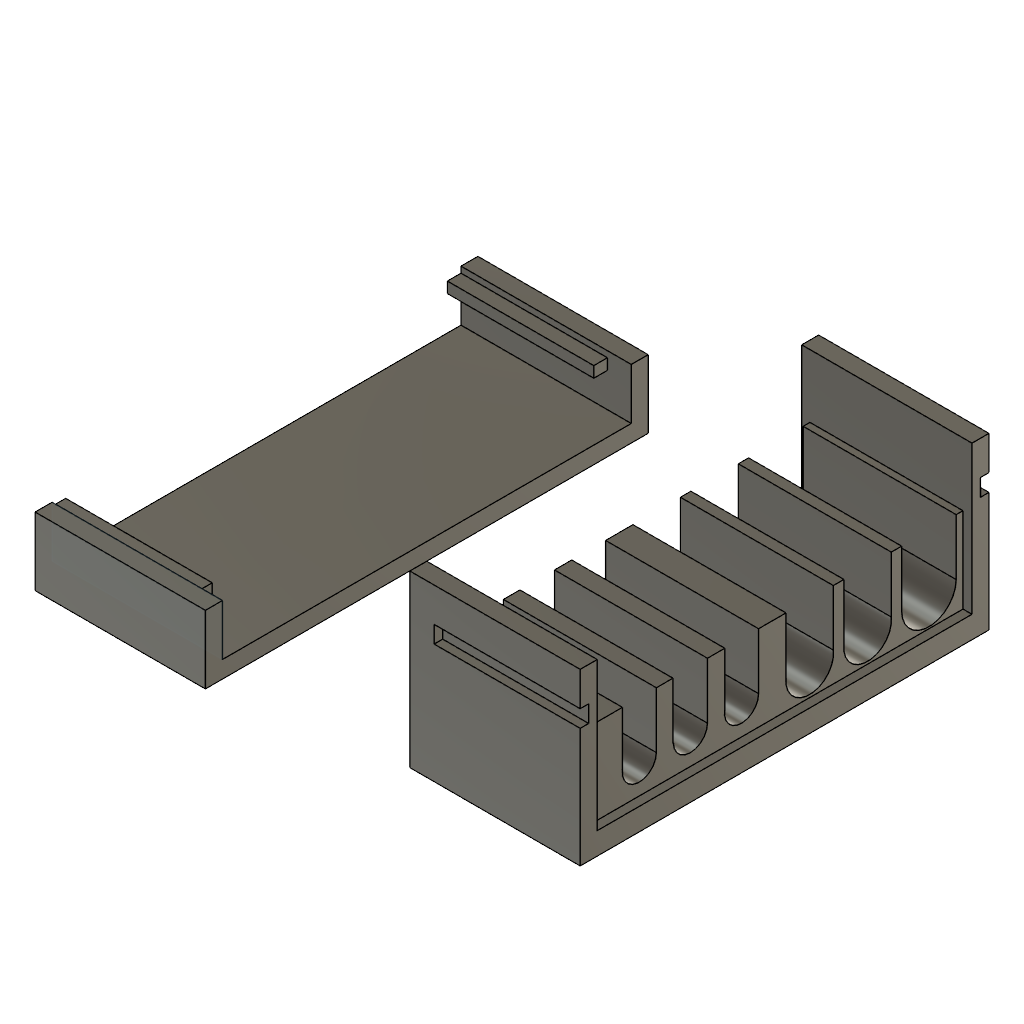
cable management clamp (Autodesk Fusion 360 design; units mm, degrees)
part number: 2026-09-18-19-42-44-531
Autodesk Fusion 360 part; units mm, degrees
note: some values were not read from the file. Set by a fixed rule: which sketch regions a step uses.
sketch "Sketch1" plane through (0, 0, 0) normal (0, 0, 1) x (1, 0, 0)
  line L0 (0, 0) -> (50, 0)
  line L1 (50, 0) -> (50, 120)
  line L2 (50, 120) -> (0, 120)
  line L3 (0, 120) -> (0, 0)
  constraint horizontal L0
  constraint vertical L1
  constraint horizontal L2
  constraint vertical L3
  constraint coincident L0.start L3.end
extrude "Extrude1" add sketch "Sketch1" along normal blind 6.5 makes body 1
sketch "Sketch2" plane through (0, 0, 6.5) normal (0, 0, 1) x (-1, 0, 0)
  line L0 (0, -120) -> (0, 0)
  line L1 (0, 0) -> (-50, 0)
  line L2 (-50, 0) -> (-50, -120)
  line L3 (-50, -120) -> (0, -120)
  line L4 (0, 0) -> (-50, 0)
  line L5 (-50, 0) -> (-50, -5)
  line L6 (-50, -5) -> (0, -5)
  line L7 (0, -5) -> (0, 0)
  constraint horizontal L4
  constraint vertical L5
  constraint horizontal L6
  constraint vertical L7
  constraint coincident L2 L5.end
  constraint coincident L0.end L1.start
extrude "Extrude2" add sketch "Sketch2" along normal blind 40 contours L0 L1 L2 L4 L5 L6 L7 bodies 1
sketch "Sketch3" plane through (0, 0, 6.5) normal (0, 0, 1) x (-1, 0, 0)
  line L0 (0, -5) -> (-50, -5)
  line L1 (-50, -5) -> (-50, -120)
  line L2 (-50, -120) -> (0, -120)
  line L3 (0, -120) -> (0, -5)
  line L4 (-50, -120) -> (0, -120)
  line L5 (0, -120) -> (0, -115)
  line L6 (0, -115) -> (-50, -115)
  line L7 (-50, -115) -> (-50, -120)
  constraint horizontal L4
  constraint vertical L5
  constraint horizontal L6
  constraint vertical L7
  constraint coincident L3 L5.end
  constraint coincident L1.end L2.start
extrude "Extrude3" add sketch "Sketch3" along normal blind 40 contours L1 L2 L3 L4 L5 L6 L7 bodies 1
sketch "Sketch4" plane through (0, 120, 0) normal (0, 1, 0) x (-1, 0, 0)
  line L0 (-50, 0) -> (0, 0)
  line L1 (0, 0) -> (0, 46.5)
  line L2 (0, 46.5) -> (-50, 46.5)
  line L3 (-50, 46.5) -> (-50, 0)
  line L4 (-50, 46.5) -> (-50, 50)
  line L5 (-50, 50) -> (0, 50)
  line L6 (0, 50) -> (0, 46.5)
  constraint coincident L2.end L3.start
  constraint perpendicular L2 L4
  constraint perpendicular L4 L5
  constraint coincident L1.end L2.start
  constraint perpendicular L5 L6
extrude "Extrude4" add sketch "Sketch4" against normal blind 5 contours L2 L4 L5 L6 bodies 1
sketch "Sketch5" plane through (0, 0, 46.5) normal (0, 0, 1) x (-1, 0, 0)
  line L0 (0, -5) -> (0, 0)
  line L1 (0, 0) -> (-50, 0)
  line L2 (-50, 0) -> (-50, -5)
  line L3 (-50, -5) -> (0, -5)
  line L4 (0, 0) -> (0, -5)
  line L5 (-50, -5) -> (-50, 0)
  constraint coincident L0.end L1.start
  constraint coincident L0.start L3.end
  constraint coincident L2.end L3.start
  constraint coincident L1.end L2.start
extrude "Extrude5" add sketch "Sketch5" along normal blind 3.5 bodies 1
sketch "Sketch6" plane through (0, 120, 0) normal (0, 1, 0) x (-1, 0, 0)
  line L0 (-50, 0) -> (0, 0)
  line L1 (0, 0) -> (0, 50)
  line L2 (0, 50) -> (-50, 50)
  line L3 (-50, 50) -> (-50, 0)
  line L4 (-50, 40) -> (0, 40)
  line L5 (0, 40) -> (0, 35)
  line L6 (0, 35) -> (-50, 35)
  line L7 (-50, 35) -> (-50, 40)
  constraint horizontal L4
  constraint vertical L5
  constraint horizontal L6
  constraint vertical L7
  constraint coincident L1 L5.end
  constraint coincident L3 L4.start
extrude "Extrude6" cut sketch "Sketch6" against normal blind 2.5 contours L1 L3 L4 L5 L6 L7 bodies 1
sketch "Sketch7" plane through (0, 0, 0) normal (0, -1, 0) x (1, 0, 0)
  line L0 (0, 0) -> (50, 0)
  line L1 (50, 0) -> (50, 50)
  line L2 (50, 50) -> (0, 50)
  line L3 (0, 50) -> (0, 0)
  line L4 (0, 40) -> (50, 40)
  line L5 (50, 40) -> (50, 35)
  line L6 (50, 35) -> (0, 35)
  line L7 (0, 35) -> (0, 40)
  constraint horizontal L4
  constraint vertical L5
  constraint horizontal L6
  constraint vertical L7
  constraint coincident L1 L5.end
  constraint coincident L3 L4.start
extrude "Extrude7" cut sketch "Sketch7" against normal blind 2.5 contours L1 L3 L4 L5 L6 L7 bodies 1
sketch "Sketch8" plane through (0, 0, 6.5) normal (0, 0, 1) x (-1, 0, 0)
  line L0 (-50, -115) -> (0, -115)
  line L1 (0, -115) -> (0, -5)
  line L2 (0, -5) -> (-50, -5)
  line L3 (-50, -5) -> (-50, -115)
  line L4 (-2.4411, -115) -> (-47.3569, -115)
  line L5 (-47.3569, -115) -> (-47.3569, -5)
  line L6 (-47.3569, -5) -> (-2.4411, -5)
  line L7 (-2.4411, -5) -> (-2.4411, -115)
  constraint horizontal L4
  constraint vertical L5
  constraint horizontal L6
  constraint vertical L7
  constraint coincident L2 L5.end
  constraint coincident L0 L4.start
extrude "Extrude8" add sketch "Sketch8" along normal blind 10 contours L0 L2 L4 L5 L6 L7 bodies 1
extrude "Extrude9" add 1 faces at (32.385, 41.6667, 16.5) along direction (0, 0, 1) blind 15 on bodies 1 bodies 1
sketch "Sketch9" plane through (2.4411, 0, 0) normal (-1, 0, 0) x (0, -1, 0)
  line L0 (-115, 6.5) -> (-5, 6.5)
  line L1 (-5, 6.5) -> (-5, 31.5)
  line L2 (-5, 31.5) -> (-115, 31.5)
  line L3 (-115, 31.5) -> (-115, 6.5)
  circle A0 centre (-105, 15) radius 8
sketch "Sketch10" plane through (2.4411, 0, 0) normal (-1, 0, 0) x (0, -1, 0)
  line L0 (-113, 15) -> (-97, 15)
  line L1 (-97, 15) -> (-97, 31.5)
  line L2 (-97, 31.5) -> (-113, 31.5)
  line L3 (-113, 31.5) -> (-113, 15)
  constraint horizontal L0
  constraint vertical L1
  constraint horizontal L2
  constraint vertical L3
extrude "Extrude10" cut sketch "Sketch10" against normal blind 70 bodies 1
extrude "Extrude11" cut sketch "Sketch9" against normal blind 70 contours A0 bodies 1
sketch "Sketch11" plane through (2.4411, 0, 0) normal (-1, 0, 0) x (0, -1, 0)
  arc A0 (-113, 15) -> (-97, 15) centre (-105, 15) ccw
  line L0 (-113, 15) -> (-113, 31.5)
  line L1 (-113, 31.5) -> (-115, 31.5)
  line L2 (-115, 31.5) -> (-115, 6.5)
  line L3 (-115, 6.5) -> (-5, 6.5)
  line L4 (-5, 6.5) -> (-5, 31.5)
  line L5 (-5, 31.5) -> (-97, 31.5)
  line L6 (-97, 31.5) -> (-97, 15)
  circle A1 centre (-87, 14.1894) radius 7
  line L7 (-93.9529, 15) -> (-80.0577, 15)
  line L8 (-80.0577, 15) -> (-80.0577, 31.5)
  line L9 (-80.0577, 31.5) -> (-93.9529, 31.5)
  line L10 (-93.9529, 31.5) -> (-93.9529, 15)
  line L11 (-234.0751, -116.6627) -> (-124.5111, -116.6627)
  line L12 (-124.5111, -116.6627) -> (-124.5111, 18.1884)
  line L13 (-124.5111, 18.1884) -> (-234.0751, 18.1884)
  line L14 (-234.0751, 18.1884) -> (-234.0751, -116.6627)
  constraint horizontal L7
  constraint vertical L8
  constraint horizontal L9
  constraint vertical L10
  constraint coincident L5 L8.end
  constraint coincident A1 L7.start
  constraint horizontal L11
  constraint vertical L12
  constraint horizontal L13
  constraint vertical L14
extrude "Extrude12" cut sketch "Sketch11" against normal blind 80 contours L5 A1 L8 L9 L10 | A1 L7 L8 | A1 L7 L8 bodies 1
sketch "Sketch12" plane through (2.4411, 0, 0) normal (-1, 0, 0) x (0, -1, 0)
  line L0 (-80.0577, 31.5) -> (-80.0577, 15.0862)
  arc A0 (-93.9529, 15) -> (-80.0577, 15.0862) centre (-87, 14.1894) ccw
  line L1 (-93.9529, 15) -> (-93.9529, 31.5)
  line L2 (-93.9529, 31.5) -> (-97, 31.5)
  line L3 (-97, 31.5) -> (-97, 15)
  arc A1 (-113, 15) -> (-97, 15) centre (-105, 15) ccw
  line L4 (-113, 15) -> (-113, 31.5)
  line L5 (-113, 31.5) -> (-115, 31.5)
  line L6 (-115, 31.5) -> (-115, 6.5)
  line L7 (-115, 6.5) -> (-5, 6.5)
  line L8 (-5, 6.5) -> (-5, 31.5)
  line L9 (-5, 31.5) -> (-80.0577, 31.5)
  circle A2 centre (-70, 14.2627) radius 7
  line L10 (-76.9514, 15.0862) -> (-63.0522, 15.0862)
  line L11 (-63.0522, 15.0862) -> (-63.0522, 31.5)
  line L12 (-63.0522, 31.5) -> (-76.9514, 31.5)
  line L13 (-76.9514, 31.5) -> (-76.9514, 15.0862)
  dimension "d25" = 14
  constraint horizontal L10
  constraint vertical L11
  constraint horizontal L12
  constraint vertical L13
  constraint coincident L9 L11.end
  constraint coincident A2 L10.start
  measures "d25" diameter of A2
extrude "Extrude13" cut sketch "Sketch12" against normal blind 80 contours L9 A2 L11 L12 L13 | A2 L10 L11 | A2 L10 L11 bodies 1
sketch "Sketch13" plane through (2.4411, 0, 0) normal (-1, 0, 0) x (0, -1, 0)
  line L0 (-63.0522, 31.5) -> (-63.0522, 15.1163)
  arc A0 (-76.9514, 15.0862) -> (-63.0522, 15.1163) centre (-70, 14.2627) ccw
  line L1 (-76.9514, 15.0862) -> (-76.9514, 31.5)
  line L2 (-76.9514, 31.5) -> (-80.0577, 31.5)
  line L3 (-80.0577, 31.5) -> (-80.0577, 15.0862)
  arc A1 (-93.9529, 15) -> (-80.0577, 15.0862) centre (-87, 14.1894) ccw
  line L4 (-93.9529, 15) -> (-93.9529, 31.5)
  line L5 (-93.9529, 31.5) -> (-97, 31.5)
  line L6 (-97, 31.5) -> (-97, 15)
  arc A2 (-113, 15) -> (-97, 15) centre (-105, 15) ccw
  line L7 (-113, 15) -> (-113, 31.5)
  line L8 (-113, 31.5) -> (-115, 31.5)
  line L9 (-115, 31.5) -> (-115, 6.5)
  line L10 (-115, 6.5) -> (-5, 6.5)
  line L11 (-5, 6.5) -> (-5, 31.5)
  line L12 (-5, 31.5) -> (-63.0522, 31.5)
  circle A3 centre (-50, 14.9754) radius 5
sketch "Sketch14" plane through (2.4411, 0, 0) normal (-1, 0, 0) x (0, -1, 0)
  line L0 (-55, 15) -> (-45.0908, 15)
  line L1 (-45.0908, 15) -> (-45.0908, 31.552)
  line L2 (-45.0908, 31.552) -> (-55, 31.552)
  line L3 (-55, 31.552) -> (-55, 15)
  constraint horizontal L0
  constraint vertical L1
  constraint horizontal L2
  constraint vertical L3
extrude "Extrude14" cut sketch "Sketch13" sketch "Sketch14" against normal blind 900 contours A3 of sketch 2 bodies 1
sketch "Sketch15" plane through (2.4411, 0, 0) normal (-1, 0, 0) x (0, -1, 0)
  line L0 (-55, 15) -> (-55, 31.5)
  line L1 (-55, 31.5) -> (-63.0522, 31.5)
  line L2 (-63.0522, 31.5) -> (-63.0522, 15.1163)
  arc A0 (-76.9514, 15.0862) -> (-63.0522, 15.1163) centre (-70, 14.2627) ccw
  line L3 (-76.9514, 15.0862) -> (-76.9514, 31.5)
  line L4 (-76.9514, 31.5) -> (-80.0577, 31.5)
  line L5 (-80.0577, 31.5) -> (-80.0577, 15.0862)
  arc A1 (-93.9529, 15) -> (-80.0577, 15.0862) centre (-87, 14.1894) ccw
  line L6 (-93.9529, 15) -> (-93.9529, 31.5)
  line L7 (-93.9529, 31.5) -> (-97, 31.5)
  line L8 (-97, 31.5) -> (-97, 15)
  arc A2 (-113, 15) -> (-97, 15) centre (-105, 15) ccw
  line L9 (-113, 15) -> (-113, 31.5)
  line L10 (-113, 31.5) -> (-115, 31.5)
  line L11 (-115, 31.5) -> (-115, 6.5)
  line L12 (-115, 6.5) -> (-5, 6.5)
  line L13 (-5, 6.5) -> (-5, 31.5)
  line L14 (-5, 31.5) -> (-45.0908, 31.5)
  line L15 (-45.0908, 31.5) -> (-45.0908, 15.9237)
  arc A3 (-54.9999, 15) -> (-45.0908, 15.9237) centre (-50, 14.9754) ccw
  line L16 (-54.9999, 15) -> (-55, 15)
  circle A4 centre (-35, 15) radius 5
  line L17 (-40, 15) -> (-29.8713, 15)
  line L18 (-29.8713, 15) -> (-29.8713, 31.5)
  line L19 (-29.8713, 31.5) -> (-40, 31.5)
  line L20 (-40, 31.5) -> (-40, 15)
  dimension "d30" = 10
  constraint horizontal L17
  constraint vertical L18
  constraint horizontal L19
  constraint vertical L20
  constraint coincident A4 L17.start
  measures "d30" diameter of A4
extrude "Extrude15" cut sketch "Sketch15" against normal blind 90 contours L14 A4 L17 L18 L19 L20 | A4 L17 | A4 L17 bodies 1
sketch "Sketch16" plane through (2.4411, 0, 0) normal (-1, 0, 0) x (0, -1, 0)
  line L0 (-29.8713, 31.5) -> (-29.8713, 15)
  line L1 (-29.8713, 15) -> (-30, 15)
  arc A0 (-40, 15) -> (-30, 15) centre (-35, 15) ccw
  line L2 (-40, 15) -> (-40, 31.5)
  line L3 (-40, 31.5) -> (-45.0908, 31.5)
  line L4 (-45.0908, 31.5) -> (-45.0908, 15.9237)
  arc A1 (-54.9999, 15) -> (-45.0908, 15.9237) centre (-50, 14.9754) ccw
  line L5 (-54.9999, 15) -> (-55, 15)
  line L6 (-55, 15) -> (-55, 31.5)
  line L7 (-55, 31.5) -> (-63.0522, 31.5)
  line L8 (-63.0522, 31.5) -> (-63.0522, 15.1163)
  arc A2 (-76.9514, 15.0862) -> (-63.0522, 15.1163) centre (-70, 14.2627) ccw
  line L9 (-76.9514, 15.0862) -> (-76.9514, 31.5)
  line L10 (-76.9514, 31.5) -> (-80.0577, 31.5)
  line L11 (-80.0577, 31.5) -> (-80.0577, 15.0862)
  arc A3 (-93.9529, 15) -> (-80.0577, 15.0862) centre (-87, 14.1894) ccw
  line L12 (-93.9529, 15) -> (-93.9529, 31.5)
  line L13 (-93.9529, 31.5) -> (-97, 31.5)
  line L14 (-97, 31.5) -> (-97, 15)
  arc A4 (-113, 15) -> (-97, 15) centre (-105, 15) ccw
  line L15 (-113, 15) -> (-113, 31.5)
  line L16 (-113, 31.5) -> (-115, 31.5)
  line L17 (-115, 31.5) -> (-115, 6.5)
  line L18 (-115, 6.5) -> (-5, 6.5)
  line L19 (-5, 6.5) -> (-5, 31.5)
  line L20 (-5, 31.5) -> (-29.8713, 31.5)
  circle A5 centre (-20, 15) radius 5.0013
  line L21 (-25.0012, 15.015) -> (-15.0406, 15.015)
  line L22 (-15.0406, 15.015) -> (-15.0406, 31.5)
  line L23 (-15.0406, 31.5) -> (-25.0012, 31.5)
  line L24 (-25.0012, 31.5) -> (-25.0012, 15.015)
  constraint horizontal L21
  constraint vertical L22
  constraint horizontal L23
  constraint vertical L24
  constraint coincident L20 L22.end
  constraint coincident A5 L21.start
extrude "Extrude16" cut sketch "Sketch16" against normal blind 900 contours L20 A5 L22 L23 L24 | A5 L21 L22 | A5 L21 L22 bodies 1
sketch "Sketch17" plane through (0, 2.5, 0) normal (0, -1, 0) x (1, 0, 0)
  line L0 (0, 35) -> (50, 35)
  line L1 (50, 35) -> (50, 40)
  line L2 (50, 40) -> (0, 40)
  line L3 (0, 40) -> (0, 35)
  line L4 (0, 40) -> (7.1471, 40)
  line L5 (7.1471, 40) -> (7.1471, 35)
  line L6 (7.1471, 35) -> (0, 35)
  line L7 (0, 35) -> (0, 40)
  constraint horizontal L4
  constraint vertical L5
  constraint horizontal L6
  constraint vertical L7
  constraint coincident L0 L5.end
  constraint coincident L2.end L3.start
extrude "Extrude17" add sketch "Sketch17" along normal blind 2.5 contours L0 L2 L3 L4 L5 L6 L7 bodies 1
sketch "Sketch18" plane through (0, 117.5, 0) normal (0, 1, 0) x (-1, 0, 0)
  line L0 (-50, 35) -> (0, 35)
  line L1 (0, 35) -> (0, 40)
  line L2 (0, 40) -> (-50, 40)
  line L3 (-50, 40) -> (-50, 35)
  line L4 (0, 35) -> (-7.0127, 35)
  line L5 (-7.0127, 35) -> (-7.0127, 40)
  line L6 (-7.0127, 40) -> (0, 40)
  line L7 (0, 40) -> (0, 35)
  constraint horizontal L4
  constraint vertical L5
  constraint horizontal L6
  constraint vertical L7
  constraint coincident L2 L5.end
  constraint coincident L0.end L1.start
extrude "Extrude18" add sketch "Sketch18" along normal blind 2.5 contours L0 L1 L2 L4 L5 L6 L7 bodies 1
sketch "Sketch19" plane through (0, 0, 0) normal (0, 0, 1) x (1, 0, 0)
sketch "Sketch20" plane through (0, 0, 0) normal (0, 0, 1) x (1, 0, 0)
sketch "Sketch21" plane through (0, 0, 0) normal (0, 0, 1) x (1, 0, 0)
  line L0 (-100, 120) -> (-50, 120)
  line L1 (-50, 120) -> (-50, -10)
  line L2 (-50, -10) -> (-100, -10)
  line L3 (-100, -10) -> (-100, 120)
  dimension "d39" = 50
  dimension "d40" = 130
  constraint horizontal L0
  constraint vertical L1
  constraint horizontal L2
  constraint vertical L3
  measures "d39" distance of L0.start L0.end
  measures "d40" distance of L0.start L2.end
sketch "Sketch22" plane through (0, 0, 0) normal (0, 0, 1) x (1, 0, 0)
  line L0 (-100, 120) -> (-50, 120)
  line L1 (-50, 120) -> (-50, 115)
  line L2 (-50, 115) -> (-100, 115)
  line L3 (-100, 115) -> (-100, 120)
  line L4 (-100, -10) -> (-50, -10)
  line L5 (-50, -10) -> (-50, -5)
  line L6 (-50, -5) -> (-100, -5)
  line L7 (-100, -5) -> (-100, -10)
  constraint horizontal L0
  constraint vertical L1
  constraint horizontal L2
  constraint vertical L3
  constraint horizontal L4
  constraint vertical L5
  constraint horizontal L6
  constraint vertical L7
extrude "Extrude19" add sketch "Sketch22" sketch "Sketch21" along normal blind 5 separate body contours L4 L5 L6 L7 of sketch 2 makes body 2
sketch "Sketch23" plane through (0, 0, 5) normal (0, 0, 1) x (-1, 0, 0)
  line L0 (100, -120) -> (100, 10)
  line L1 (100, 10) -> (50, 10)
  line L2 (50, 10) -> (50, -120)
  line L3 (50, -120) -> (100, -120)
  line L4 (100, 10) -> (50, 10)
  line L5 (50, 10) -> (50, 5)
  line L6 (50, 5) -> (100, 5)
  line L7 (100, 5) -> (100, 10)
  line L8 (100, -120) -> (50, -120)
  line L9 (50, -120) -> (50, -115)
  line L10 (50, -115) -> (100, -115)
  line L11 (100, -115) -> (100, -120)
  constraint horizontal L4
  constraint vertical L5
  constraint horizontal L6
  constraint vertical L7
  constraint coincident L2 L5.end
  constraint coincident L0.end L1.start
  constraint horizontal L8
  constraint vertical L9
  constraint horizontal L10
  constraint vertical L11
  constraint coincident L2 L9.end
  constraint coincident L0.start L3.end
extrude "Extrude20" add sketch "Sketch23" along normal blind 15 contours L0 L1 L2 L4 L5 L6 L7 bodies 2
sketch "Sketch24" plane through (0, 0, 5) normal (0, 0, 1) x (-1, 0, 0)
  line L0 (100, 5) -> (50, 5)
  line L1 (50, 5) -> (50, -120)
  line L2 (50, -120) -> (100, -120)
  line L3 (100, -120) -> (100, 5)
  line L4 (100, -120) -> (50, -120)
  line L5 (50, -120) -> (50, -115)
  line L6 (50, -115) -> (100, -115)
  line L7 (100, -115) -> (100, -120)
  constraint horizontal L4
  constraint vertical L5
  constraint horizontal L6
  constraint vertical L7
  constraint coincident L1 L5.end
  constraint coincident L2.end L3.start
extrude "Extrude21" add sketch "Sketch24" along normal blind 15 contours L1 L2 L3 L4 L5 L6 L7 bodies 2
sketch "Sketch25" plane through (0, 115, 0) normal (0, -1, 0) x (1, 0, 0)
  line L0 (-100, 5) -> (-50, 5)
  line L1 (-50, 5) -> (-50, 20)
  line L2 (-50, 20) -> (-100, 20)
  line L3 (-100, 20) -> (-100, 5)
  line L4 (-100, 15) -> (-50, 15)
  line L5 (-50, 15) -> (-50, 18.2038)
  line L6 (-50, 18.2038) -> (-100, 18.2038)
  line L7 (-100, 18.2038) -> (-100, 15)
  constraint horizontal L4
  constraint vertical L5
  constraint horizontal L6
  constraint vertical L7
  constraint coincident L1 L5.end
  constraint coincident L3 L4.start
extrude "Extrude22" add sketch "Sketch25" along normal blind 4 contours L1 L3 L4 L5 L6 L7 bodies 2
sketch "Sketch26" plane through (0, -5, 0) normal (0, 1, 0) x (-1, 0, 0)
  line L0 (50, 5) -> (100, 5)
  line L1 (100, 5) -> (100, 20)
  line L2 (100, 20) -> (50, 20)
  line L3 (50, 20) -> (50, 5)
sketch "Sketch27" plane through (0, -5, 0) normal (0, 1, 0) x (-1, 0, 0)
sketch "Sketch28" plane through (0, -5, 0) normal (0, 1, 0) x (-1, 0, 0)
  line L0 (50, 15) -> (100, 15)
  line L1 (100, 15) -> (100, 19)
  line L2 (100, 19) -> (50, 19)
  line L3 (50, 19) -> (50, 15)
  dimension "d49" = 50
  dimension "d50" = 4
  constraint horizontal L0
  constraint vertical L1
  constraint horizontal L2
  constraint vertical L3
  measures "d49" distance of L0.start L0.end
  measures "d50" distance of L0.start L2.end
extrude "Extrude23" add sketch "Sketch28" along normal blind 4 bodies 2
sketch "Sketch29" plane through (0, 111, 0) normal (0, -1, 0) x (1, 0, 0)
  line L0 (-100, 18.2038) -> (-100, 15)
  line L1 (-100, 15) -> (-50, 15)
  line L2 (-50, 15) -> (-50, 18.2038)
  line L3 (-50, 18.2038) -> (-100, 18.2038)
  line L4 (-50, 18.2038) -> (-57, 18.2038)
  line L5 (-57, 18.2038) -> (-57, 15)
  line L6 (-57, 15) -> (-50, 15)
  line L7 (-50, 15) -> (-50, 18.2038)
  dimension "d53" = 7
  constraint horizontal L4
  constraint vertical L5
  constraint horizontal L6
  constraint vertical L7
  constraint coincident L2.end L3.start
  measures "d53" distance of L2.end L4.end
extrude "Extrude24" cut sketch "Sketch29" against normal blind 4 contours L1 L2 L3 L4 L5 L6 L7 bodies 2
sketch "Sketch30" plane through (0, -1, 0) normal (0, 1, 0) x (-1, 0, 0)
  line L0 (50, 19) -> (50, 15)
  line L1 (50, 15) -> (100, 15)
  line L2 (100, 15) -> (100, 19)
  line L3 (100, 19) -> (50, 19)
  line L4 (50, 15) -> (57, 15)
  line L5 (57, 15) -> (57, 19)
  line L6 (57, 19) -> (50, 19)
  line L7 (50, 19) -> (50, 15)
  dimension "d56" = 7
  constraint horizontal L4
  constraint vertical L5
  constraint horizontal L6
  constraint vertical L7
  constraint coincident L0.end L1.start
  measures "d56" distance of L0.end L4.end
extrude "Extrude25" cut sketch "Sketch30" against normal blind 4 contours L0 L1 L3 L4 L5 L6 L7 bodies 2
equation "d15 = cm"
